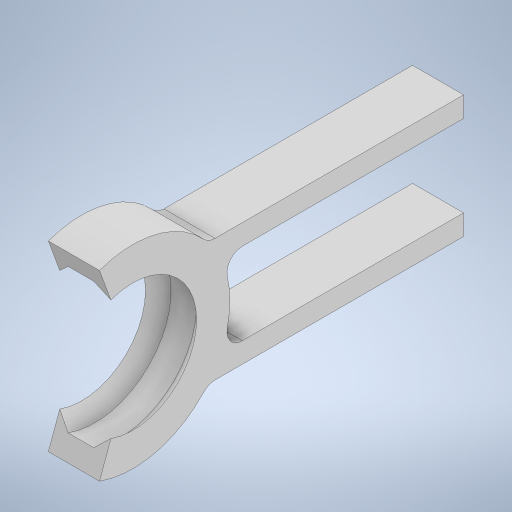
# Autodesk Inventor part: 6mm lens mount
Saved by Autodesk Inventor 2024 (Build 280153000, 153)
## iProperties
Created: 2024-11-13
Part Number: 6mm lens mount
Material: Generic
Document SubType Name: Modeling
Designer: Williamow
Density: 1 g/cm^3
Appearance: Default
Author: Williamow
Autodesk Inventor part; units mm, degrees
ref_plane "YZ Plane" through (0, 0, 0) normal (1, 0, 0) x (0, 1, 0)
ref_plane "XZ Plane" through (0, 0, 0) normal (0, 1, 0) x (-1, 0, 0)
ref_plane "XY Plane" through (0, 0, 0) normal (0, 0, 1) x (1, 0, 0)
sketch "Sketch4" plane through (0, 0, 0) normal (0, 1, 0) x (-1, 0, 0)
  line L0 (1, -2.5) -> (1, -3.8)
  line L1 (1, -3.8) -> (-1, -3.8)
  line L2 (-1, -3.8) -> (-1, -2.5)
  line L3 (-1, -2.5) -> (-0.5, -3)
  line L4 (-0.5, -3) -> (0.5, -3)
  line L5 (0.5, -3) -> (1, -2.5)
  line L6 (0, 0) -> (-1.4783, 0)
  point P0 (0, -3)
  dimension "d21" = 1
  dimension "d22" = 3
  dimension "d24" = 0.8
  dimension "d32" = 0.5
  constraints: 14 end point, 3 perpendicular, 2 equal length, 1 horizontal, 1 midpoint, 1 parallel, 1 vertical, 1 vertical alignment
  measures "d21" distance of L3.end L4.end
  measures "d22" distance from line of L6.start L4
  measures "d24" distance between parallel lines of L1 L4
  measures "d32" distance from line of L0.start L4
revolve "Revolution1" add sketch "Sketch4" angle 220 mid plane about axis through (0, 0, 0) along (1, 0, 0)
sketch "Sketch5" plane through (1, 0, 0) normal (1, 0, 0) x (0, 0, -1)
  arc A0 (-1.2997, -3.5708) -> (-1.2997, 3.5708) centre (0, 0) ccw projected
  line L0 (2.9462, -2.4) -> (12.9462, -2.4)
  line L1 (12.9462, -2.4) -> (12.9462, -1.6)
  line L2 (12.9462, -1.6) -> (3.4467, -1.6)
  line L3 (3.4467, 1.6) -> (12.9462, 1.6)
  line L4 (12.9462, 1.6) -> (12.9462, 2.4)
  line L5 (12.9462, 2.4) -> (2.9462, 2.4)
  point P0 (0, 0)
  point P1 (12.9462, 2)
  point P2 (12.9462, -2)
  dimension "d26" = 0.8
  dimension "d27" = 10
  dimension "d28" = 4
  dimension "d10" = 1.5
  dimension "d11" = 0.8
  dimension "d12" = 6
  dimension "d13" = 5.5
  dimension "d14" = 0.5
  dimension "d15" = 0.8
  dimension "d16" = 8
  constraints: 12 end point, 4 point on circle, 3 perpendicular, 2 equal length, 2 midpoint, 2 point on line, 1 horizontal, 1 parallel
  measures "d26" distance of L0.end L1.end
  measures "d27" distance of L0.start L0.end
  measures "d28" distance of point (12.946, 2) point (12.946, -2)
extrude "Extrusion5" add sketch "Sketch5" against normal up to surface (2 mm away)
fillet "Fillet1" radius 0.6 4 edges at (0, 2.4, -2.9462) (0, 1.6, -3.4467) (0, -1.6, -3.4467) (0, -2.4, -2.9462)
sketch "Sketch1" plane through (0, 0, 0) normal (0, 1, 0) x (-1, 0, 0)
  line L0 (-1, 2.3) -> (0, 3.3)
  line L1 (0, 3.3) -> (1, 2.3)
  line L2 (1, 2.3) -> (1, 4.5)
  line L3 (1, 4.5) -> (-1, 4.5)
  line L4 (-1, 4.5) -> (-1, 2.3)
  line L5 (0, 0) -> (-2.1371, 0)
  line L6 (-1, -2.3) -> (0, -3.3)
  line L7 (0, -3.3) -> (1, -2.3)
  line L8 (1, -2.3) -> (1, -4.5)
  line L9 (1, -4.5) -> (-1, -4.5)
  line L10 (-1, -4.5) -> (-1, -2.3)
  dimension "d0" = 45
  dimension "d1" = 3.3
  dimension "d2" = 2
  dimension "d3" = 4.5
  constraints: 22 end point, 5 symmetric about line, 4 perpendicular, 1 horizontal, 1 vertical, 1 vertical alignment
  measures "d0" angle of L4 L0
  measures "d1" distance of L5.start L0.end
  measures "d2" distance of L2.end L3.end
  measures "d3" vertical distance of L2.end L5.start
sketch "Sketch2" plane through (-1, 0, 4.5) normal (0, 0, 1) x (1, 0, 0)
  line L0 (0, 0) -> (2, 0) projected
  line L1 (2, 0) -> (2, -2)
  line L2 (2, -2) -> (-3, -2)
  line L3 (-3, -2) -> (0, 0)
  point P0 (1, 0)
  dimension "d6" = 2
  dimension "d7" = 5
  constraints: 6 end point, 1 perpendicular, 1 vertical
  measures "d6" distance of L0.end L1.end
  measures "d7" distance of L1.end L2.end
body "Solid1"
body "Solid2"
body "Solid3"
